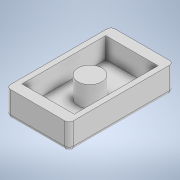
# Autodesk Inventor part: TestPart
Saved by Autodesk Inventor 2021 (Build 250183000, 183)
## iProperties
Created: 2022-05-25
Part Number: TestPart
Material: Generic
Document SubType Name: Modeling
Designer: cmzgt
Density: 1 g/cm^3
Appearance: Default
Author: cmzgt
Autodesk Inventor part; units mm, degrees
ref_plane "YZ Plane" through (0, 0, 0) normal (1, 0, 0) x (0, 1, 0)
ref_plane "XZ Plane" through (0, 0, 0) normal (0, 1, 0) x (-1, 0, 0)
ref_plane "XY Plane" through (0, 0, 0) normal (0, 0, 1) x (1, 0, 0)
sketch "Sketch1" plane through (0, 0, 0) normal (0, 1, 0) x (-1, 0, 0)
  line L0 (-38.1, 63.5) -> (38.1, 63.5)
  line L1 (38.1, 63.5) -> (38.1, -63.5)
  line L2 (38.1, -63.5) -> (-38.1, -63.5)
  line L3 (-38.1, -63.5) -> (-38.1, 63.5)
  line L4 (-38.1, 63.5) -> (38.1, -63.5) construction
  line L5 (38.1, 63.5) -> (-38.1, -63.5) construction
  line L6 (-31.75, -50.8) -> (31.75, -50.8)
  line L7 (31.75, -50.8) -> (31.75, 50.8)
  line L8 (31.75, 50.8) -> (-31.75, 50.8)
  line L9 (-31.75, 50.8) -> (-31.75, -50.8)
  line L10 (-31.75, -50.8) -> (31.75, 50.8) construction
  line L11 (31.75, -50.8) -> (-31.75, 50.8) construction
  point P0 (0, 0)
  dimension "d0" = 76.2
  dimension "d1" = 127
  dimension "d2" = 63.5
  dimension "d3" = 101.6
  constraints: 24 end point, 4 midpoint, 4 parallel, 2 horizontal, 2 perpendicular
  measures "d0" distance of L1.end L2.end
  measures "d1" distance of L0.end L1.end
  measures "d2" distance of L8.end L7.end
  measures "d3" distance of L7.end L6.end
extrude "Extrusion1" add sketch "Sketch1" along normal blind 25.4
sketch "Sketch2" plane through (0, 0, 0) normal (0, -1, 0) x (1, 0, 0)
  line L0 (-38.1, 63.5) -> (38.1, 63.5) projected
  line L1 (38.1, -63.5) -> (-38.1, -63.5) projected
  line L2 (38.1, 63.5) -> (-38.1, 63.5)
  line L3 (-38.1, 63.5) -> (-38.1, -63.5)
  line L4 (-38.1, -63.5) -> (38.1, -63.5)
  line L5 (38.1, -63.5) -> (38.1, 63.5)
  point P0 (0, 0)
  constraints: 8 end point, 2 parallel, 1 horizontal, 1 perpendicular
extrude "Extrusion2" add sketch "Sketch2" along normal blind 6.35
fillet "Fillet1" radius 5.08 4 edges at (38.1, -6.35, 0) (0, -6.35, -63.5) (-38.1, -6.35, 0) (0, -6.35, 63.5)
fillet "Fillet2" radius 5.08 8 edges at (36.6121, -4.8621, -62.0121) (38.1, 12.065, -63.5) (-36.6121, -4.8621, -62.0121) (-38.1, 12.065, -63.5) (36.6121, -4.8621, 62.0121) (38.1, 12.065, 63.5) (-36.6121, -4.8621, 62.0121) (-38.1, 12.065, 63.5)
sketch "Sketch3" plane through (0, 0, 0) normal (0, 1, 0) x (1, 0, 0)
  circle A0 centre (0, 0) radius 14.5196
  constraints: 1 centre point, 1 coincident
extrude "Extrusion3" add sketch "Sketch3" along normal up to surface (25.4 mm away)
body "Solid1"
